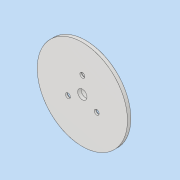
# Autodesk Inventor part: SmallSpoolEndAft
Saved by Autodesk Inventor 2017.3 (Build 213256000, 256)
## iProperties
Created: 2018-04-03
Part Number: SmallSpoolEndAft
Material: ABS Plastic
Document SubType Name: Modeling
Designer: Derek Wider
Density: 1.06 g/cm^3
Appearance: Smooth - White
Author: Derek Wider
Autodesk Inventor part; units mm, degrees
ref_plane "YZ Plane" through (0, 0, 0) normal (1, 0, 0) x (0, 1, 0)
ref_plane "XZ Plane" through (0, 0, 0) normal (0, 1, 0) x (-1, 0, 0)
ref_plane "XY Plane" through (0, 0, 0) normal (0, 0, 1) x (1, 0, 0)
sketch "Sketch1" plane through (0, 0, 0) normal (0, 0, 1) x (1, 0, 0)
  circle A0 centre (0, 0) radius 33.655
  dimension "d0" = 67.31
  constraints: 1 centre point, 1 coincident
  measures "d0" diameter of A0
extrude "Extrusion1" add sketch "Sketch1" along normal blind 2.54
sketch "Sketch2" plane through (0, 0, 0) normal (0, 0, -1) x (-1, 0, 0)
  circle A0 centre (0, 12.3825) radius 1.8415
  point P0 (0, 0)
  dimension "d3" = 3.683
  dimension "d4" = 12.3825
  constraints: 1 centre point
  measures "d3" diameter of A0
  measures "d4" distance of point (0, 0) A0.centre
extrude "Extrusion2" cut sketch "Sketch2" against normal through all
chamfer "Chamfer1" distance 1.27 angle 45 1 edges at (1.8415, 12.3825, 0)
pattern_circular "Circular Pattern1" count 3 over 360 about axis through (0, 0, 0) along (0, 0, 1) of "Extrusion2", "Chamfer1"
sketch "Sketch3" plane through (0, 0, 0) normal (0, 0, -1) x (-1, 0, 0)
  circle A0 centre (0, 0) radius 3.4925
  circle A1 centre (0, 0) radius 4.8641
  line L0 (0, 0) -> (9.525, 5.4993) construction
  line L1 (0, 0) -> (10.9985, 0) construction
  circle A2 centre (9.525, 5.4993) radius 1.27
  circle A3 centre (9.525, 5.4993) radius 3.175
  line L2 (0, 0) -> (-9.525, 5.4993) construction
  line L3 (0, 0) -> (10.9985, 0) construction
  line L4 (0, 0) -> (0, -10.9985) construction
  circle A4 centre (-9.525, 5.4993) radius 1.27
  circle A5 centre (-9.525, 5.4993) radius 3.175
  circle A6 centre (0, -10.9985) radius 1.27
  circle A7 centre (0, -10.9985) radius 3.175
  arc A8 (-8.5725, 8.528) -> (8.5725, 8.528) centre (0, 35.7868) ccw
  arc A9 (11.6717, 3.16) -> (3.0992, -11.688) centre (30.9923, -17.8934) ccw
  arc A10 (-3.0992, -11.688) -> (-11.6717, 3.16) centre (-30.9923, -17.8934) ccw
  dimension "d13" = 6.985
  dimension "d14" = 9.7282
  dimension "d15" = 30
  dimension "d16" = 2.54
  dimension "d17" = 6.35
  dimension "d18" = 150
  dimension "d19" = 19.05
  dimension "d20" = 28.575
  constraints: 12 point on circle, 11 centre point, 10 end point, 8 coincident, 6 equal radius, 6 tangent, 4 equal length, 2 horizontal, 1 vertical
  measures "d13" diameter of A0
  measures "d14" diameter of A1
  measures "d15" angle of L1 L0
  measures "d16" diameter of A2
  measures "d17" diameter of A3
  measures "d18" angle of L3 L2
  measures "d19" distance of L4.end L0.end
  measures "d20" radius of A9
extrude "Extrusion3" add sketch "Sketch3" along normal blind 8.89 contours A3 | A3 A9 A7 A10 A5 A8 | A5 | A7
extrude "Extrusion4" cut sketch "Sketch3" against normal through all contours A0
sketch "Sketch4" plane through (0, 0, 0) normal (1, 0, 0) x (0, 1, 0)
  line L0 (10.541, -10.0385) -> (19.3172, -3.8934)
  line L1 (19.3172, -3.8934) -> (19.3172, -10.0385)
  line L2 (19.3172, -10.0385) -> (10.541, -10.0385)
  line L3 (33.655, 2.54) -> (-33.655, 2.54) construction
  line L4 (0, 2.54) -> (0, 18.6348) construction
  point P0 (0, 0)
  dimension "d25" = 10.541
  dimension "d26" = 35
  constraints: 8 end point, 2 vertical, 1 midpoint, 1 perpendicular
  measures "d25" distance from line of L4 L0.start
  measures "d26" angle of L2 L0
revolve "Revolution1" cut sketch "Sketch4" angle 360 about axis through (0, 0, 2.54) along (0, 0, 1)
sketch "Sketch5" plane through (0, 0, -8.89) normal (0, 0, -1) x (-1, 0, 0)
  circle A0 centre (0, 0) radius 6.4643
  dimension "d28" = 12.9286
  constraints: 1 centre point, 1 coincident
  measures "d28" diameter of A0
extrude "Extrusion5" cut sketch "Sketch5" against normal blind 1.905
body "Solid1"
